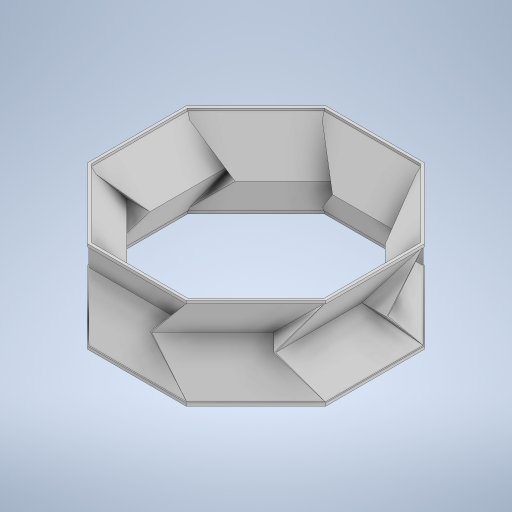
# Autodesk Inventor part: 팔각형 OV-PAM 층 한개
Saved by Autodesk Inventor 2024 (Build 280153000, 153)
## iProperties
Created: 2023-06-16
Part Number: 팔각형 OV-PAM 층 한개
Material: 일반
Document SubType Name: Modeling
Designer: jsw
Density: 1 g/cm^3
Appearance: 기본값
Author: jsw
Autodesk Inventor part; units mm, degrees
ref_plane "YZ Plane" through (0, 0, 0) normal (1, 0, 0) x (0, 1, 0)
ref_plane "XZ Plane" through (0, 0, 0) normal (0, 1, 0) x (-1, 0, 0)
ref_plane "XY Plane" through (0, 0, 0) normal (0, 0, 1) x (1, 0, 0)
sketch "스케치1" plane through (0, 0, 0) normal (0, 1, 0) x (-1, 0, 0)
  line L0 (-32.5919, 13.5) -> (-13.5, 32.5919)
  line L1 (-13.5, 32.5919) -> (13.5, 32.5919)
  line L2 (13.5, 32.5919) -> (32.5919, 13.5)
  line L3 (32.5919, 13.5) -> (32.5919, -13.5)
  line L4 (32.5919, -13.5) -> (13.5, -32.5919)
  line L5 (13.5, -32.5919) -> (-13.5, -32.5919)
  line L6 (-13.5, -32.5919) -> (-32.5919, -13.5)
  line L7 (-32.5919, -13.5) -> (-32.5919, 13.5)
  line L8 (-13.7071, 33.0919) -> (13.7071, 33.0919)
  line L9 (13.7071, 33.0919) -> (33.0919, 13.7071)
  line L10 (33.0919, 13.7071) -> (33.0919, -13.7071)
  line L11 (33.0919, -13.7071) -> (13.7071, -33.0919)
  line L12 (13.7071, -33.0919) -> (-13.7071, -33.0919)
  line L13 (-13.7071, -33.0919) -> (-33.0919, -13.7071)
  line L14 (-33.0919, -13.7071) -> (-33.0919, 13.7071)
  line L15 (-33.0919, 13.7071) -> (-13.7071, 33.0919)
  point P0 (0, 0)
  point P1 (0, 0)
  point P2 (0, 0)
  dimension "d0" = 27
  dimension "d2" = 0.5
  constraints: 32 end point, 2 coincident, 2 horizontal, 34 other
  measures "d0" distance of L0.end L1.end
  measures "d2" distance between parallel lines of L10 L3
extrude "돌출2" add sketch "스케치1" along normal blind 12 contours L0 L1 L2 L3 L4 L5 L6 L7 | L8 L9 L10 L11 L12 L13 L14 L15
ref_plane "작업 평면2" through (33.0919, 0, 13.7071) normal (-0.8660254, -0.5, 0) x (0, 0, -1)
sketch "스케치3" plane through (33.0919, 0, 13.7071) normal (1, 0, 0) x (0, 0, -1)
  line L0 (0, 0) -> (0, 12) projected
  line L1 (0, 12) -> (27.4142, 12) projected
  line L2 (0, 0) -> (27.4142, 0)
  line L3 (27.4142, 0) -> (27.4142, 12)
  line L4 (27.4142, 12) -> (0, 12)
  line L5 (0, 12) -> (0, 0)
  line L6 (0, 12) -> (-7.3047, 12)
  line L7 (-19.3848, 12) -> (0, 12) projected
  line L8 (0, 0) -> (-7.3047, 12)
  line L9 (27.4142, 12) -> (13.7071, 12)
  line L10 (17.2071, 12) -> (27.4142, 0)
  point P0 (13.7071, 0)
  point P1 (17.2071, 12)
  dimension "d17" = 121.33
  dimension "d49" = 3.5
  constraints: 16 end point, 5 midpoint, 2 parallel, 2 point on line, 1 horizontal, 1 perpendicular
  measures "d17" angle of L8 L2
  measures "d49" distance of point (13.707, 12) L10.start
extrude "돌출4" cut sketch "스케치3" against normal up to surface contours L8 L6 L0 | L0 L1 L10 L2 surface through (33.0919, 0, 13.7071) normal (-0.8660254, -0.5, 0)
pattern_circular "원형 패턴1" count 8 over 360 about axis through (0, -10, 0) along (0, 1, 0) of "돌출4"
mirror "미러5" about plane through (0, 12, 0) normal (0, 1, 0) of "돌출2", "돌출4", "원형 패턴1"
sketch "스케치9" plane through (-13.7071, 24, -33.0919) normal (0, 1, 0) x (1, 0, 0)
  line L0 (46.799, -46.799) -> (46.799, -19.3848) projected
  line L1 (46.799, -19.3848) -> (27.4142, 0) projected
  line L2 (27.4142, 0) -> (0, 0) projected
  line L3 (0, 0) -> (-19.3848, -19.3848) projected
  line L4 (-19.3848, -19.3848) -> (-19.3848, -46.799) projected
  line L5 (-19.3848, -46.799) -> (0, -66.1838) projected
  line L6 (0, -66.1838) -> (27.4142, -66.1838) projected
  line L7 (27.4142, -66.1838) -> (46.799, -46.799) projected
  point P0 (13.7071, -33.0919)
extrude "돌출8" add sketch "스케치9" along normal blind 0.8
sketch "스케치10" plane through (0, 0, 0) normal (0, -1, 0) x (1, 0, 0)
  line L0 (33.0919, 13.7071) -> (33.0919, -13.7071) projected
  line L1 (13.7071, 33.0919) -> (33.0919, 13.7071) projected
  line L2 (-13.7071, 33.0919) -> (13.7071, 33.0919) projected
  line L3 (-33.0919, 13.7071) -> (-13.7071, 33.0919) projected
  line L4 (-33.0919, -13.7071) -> (-33.0919, 13.7071) projected
  line L5 (-13.7071, -33.0919) -> (-33.0919, -13.7071) projected
  line L6 (13.7071, -33.0919) -> (-13.7071, -33.0919) projected
  line L7 (33.0919, -13.7071) -> (13.7071, -33.0919) projected
  point P0 (0, 0)
extrude "돌출9" add sketch "스케치10" along normal blind 0.8
shell "쉘6" thickness 0.5 removed faces 2 at (4.569, 24.8, 11.0306) at (-11.0306, -0.8, -4.569)
sketch "스케치12" plane through (-13.7071, 24.8, -33.0919) normal (0, 1, 0) x (1, 0, 0)
  line L0 (46.299, -19.5919) -> (46.299, -46.5919) projected
  line L1 (46.299, -46.5919) -> (27.2071, -65.6838) projected
  line L2 (27.2071, -65.6838) -> (0.2071, -65.6838) projected
  line L3 (0.2071, -65.6838) -> (-18.8848, -46.5919) projected
  line L4 (-18.8848, -46.5919) -> (-18.8848, -19.5919) projected
  line L5 (-18.8848, -19.5919) -> (0.2071, -0.5) projected
  line L6 (0.2071, -0.5) -> (27.2071, -0.5) projected
  line L7 (27.2071, -0.5) -> (46.299, -19.5919) projected
  line L8 (46.799, -19.3848) -> (27.4142, 0) projected
  line L9 (27.4142, 0) -> (0, 0) projected
  line L10 (0, 0) -> (-19.3848, -19.3848) projected
  line L11 (-19.3848, -19.3848) -> (-19.3848, -46.799) projected
  line L12 (-19.3848, -46.799) -> (0, -66.1838) projected
  line L13 (0, -66.1838) -> (27.4142, -66.1838) projected
  line L14 (27.4142, -66.1838) -> (46.799, -46.799) projected
  line L15 (46.799, -46.799) -> (46.799, -19.3848) projected
  line L16 (-0.1243, 0.3) -> (27.5385, 0.3)
  line L17 (27.5385, 0.3) -> (47.099, -19.2605)
  line L18 (47.099, -19.2605) -> (47.099, -46.9233)
  line L19 (47.099, -46.9233) -> (27.5385, -66.4838)
  line L20 (27.5385, -66.4838) -> (-0.1243, -66.4838)
  line L21 (-0.1243, -66.4838) -> (-19.6848, -46.9233)
  line L22 (-19.6848, -46.9233) -> (-19.6848, -19.2605)
  line L23 (-19.6848, -19.2605) -> (-0.1243, 0.3)
  point P0 (13.7071, -33.0919)
  point P1 (13.7071, -33.0919)
  dimension "d50" = 0.3
  constraints: 16 end point, 1 coincident, 1 horizontal, 17 other
  measures "d50" distance between parallel lines of L9 L16
extrude "돌출10" add sketch "스케치12" against normal blind 0.8 contours L16 L17 L18 L19 L20 L21 L22 L23
ref_plane "작업 평면6" through (-13.7071, 12, -33.0919) normal (0, 1, 0) x (1, 0, 0)
mirror "미러8" about plane through (-13.7071, 12, -33.0919) normal (0, 1, 0) of "돌출10"
